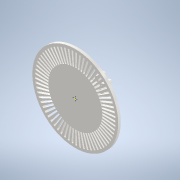
# Autodesk Inventor part: 正齿轮1
Saved by Autodesk Inventor 2020 (Build 240168000, 168)
## iProperties
CustomPartVersion: 1
Created: 2019-06-21
Part Number: 正齿轮1
Material: Steel
Document SubType Name: Modeling
Designer: User
Categories: <?xml version="1.0" encoding="UTF-16"?> <MemberInstance><Categories><FamilyTemplate><FamilyTemplateParameter ValueType="xs:double" Id="1" ObjectReferenceKey="da_z" ObjectType="kUserParameterObject"/><FamilyTemplateParameter ValueType="xs:double" Id="2" ObjectReferenceKey="da_b" ObjectType="kUserParameterObject"/><FamilyTemplateParameter ValueType="xs:double" Id="3" ObjectReferenceKey="da_beta" ObjectType="kUserParameterObject"/><FamilyTemplateParameter ValueType="xs:double" Id="4" ObjectReferenceKey="da_da" ObjectType="kUserParameterObject"/><FamilyTemplateParameter ValueType="xs:double" Id="5" ObjectReferenceKey="da_aw" ObjectType="kUserParameterObject"/><FamilyTemplateParameter ValueType="xs:string" Id="6" ObjectReferenceKey="EAIAABAAAACIAQAAAAAAAIAAAAAAAAAA" ObjectType="83910656" SubObjectId="SurfaceGeometry"/></FamilyTemplate><ParamToTemplateMap><ParamToTemplate CategoryParameter="//CategoryParameter[@InternalName='046C89C9-8512-4d59-83FE-43B91F4F132A']" TemplateParameter="1"/><ParamToTemplate CategoryParameter="//CategoryParameter[@InternalName='2552DF32-E462-4b46-AEBF-C6C7768E72AC']" TemplateParameter="2"/><ParamToTemplate CategoryParameter="//CategoryParameter[@InternalName='C9EE641D-15FC-4fae-A226-E94C4372FDD7']" TemplateParameter="3"/><ParamToTemplate><ParamToTemplate CategoryParameter="//CategoryParameter[@InternalName='00B6519A-459B-49c7-AD84-2E56D39A5744']" ConstantValue="0.104000"/></ParamToTemplate><ParamToTemplate><ParamToTemplate CategoryParameter="//CategoryParameter[@InternalName='04B31F0E-C7A6-4894-AA32-9629BEFACF47']" ConstantValue="1.000000"/></ParamToTemplate><ParamToTemplate><ParamToTemplate CategoryParameter="//CategoryParameter[@InternalName='43CBEC2E-7847-49e7-A936-2F7889FCB2D9']" ConstantValue="0.250000"/></ParamToTemplate><ParamToTemplate><ParamToTemplate CategoryParameter="//CategoryParameter[@InternalName='B1EFC894-105D-4ebd-86BF-FA20ED196853']" ConstantValue="0.333500"/></ParamToTemplate><ParamToTemplate><ParamToTemplate CategoryParameter="//CategoryParameter[@InternalName='51175063-3D10-4879-93E8-6246FE8B403D']" ConstantValue="2060000000.000000"/></ParamToTemplate><ParamToTemplate><ParamToTemplate CategoryParameter="//CategoryParameter[@InternalName='A3A52E27-4454-46a9-B0BD-C932399B70AF']" ConstantValue="0.300000"/></ParamToTemplate><ParamToTemplate><ParamToTemplate CategoryParameter="//CategoryParameter[@InternalName='91B76062-C214-41d9-B1B9-14D2AB99603D']" ConstantValue="0.080000"/></ParamToTemplate><ParamToTemplate><ParamToTemplate CategoryParameter="//CategoryParameter[@InternalName='374E806E-8B8A-4dda-A9AA-1039D6500AD2']" ConstantValue="12.500000"/></ParamToTemplate><ParamToTemplate><ParamToTemplate CategoryParameter="//CategoryParameter[@InternalName='2D373A89-B862-43d6-8D0B-0CBF12AB9F6C']" ConstantValue="0.349066"/></ParamToTemplate><ParamToTemplate CategoryParameter="//CategoryParameter[@InternalName='37777632-D6A2-4fac-9D53-DB8ACD95C989']" TemplateParameter="4"/><ParamToTemplate CategoryParameter="//CategoryParameter[@InternalName='FD1017F1-B727-4f7e-9707-0F86F1FF9423']" TemplateParameter="5"/><ParamToTemplate><ParamToTemplate CategoryParameter="//CategoryParameter[@InternalName='9E1B4470-B2D3-4ff1-B813-535BB4CDF51A']" ConstantValue="3520000.000000"/></ParamToTemplate><ParamToTemplate><ParamToTemplate CategoryParameter="//CategoryParameter[@InternalName='F8452263-BFF6-458c-9FB1-07C4B99E95CD']" ConstantValue="11400000.000000"/></ParamToTemplate><ParamToTemplate><ParamToTemplate CategoryParameter="//CategoryParameter[@InternalName='3E3BB259-FD49-497f-8171-6EBC954A3479']" ConstantValue="2.000000"/></ParamToTemplate><ParamToTemplate CategoryParameter="//CategoryParameter[@InternalName='27C3BAF2-7550-4e4b-AE2C-0DB134B7D9B7']" TemplateParameter="6"/></ParamToTemplateMap><Category DisplayName="Gear" InternalName="DC85795E-93AB-48d5-8EEE-5A27447B64BD" Mnemonic="Gear"><CategoryParameter DisplayName="z" InternalName="046C89C9-8512-4d59-83FE-43B91F4F132A" Mnemonic="z"/><CategoryParameter DisplayName="b" InternalName="2552DF32-E462-4b46-AEBF-C6C7768E72AC" Mnemonic="b"/><CategoryParameter DisplayName="||b|" InternalName="C9EE641D-15FC-4fae-A226-E94C4372FDD7" Mnemonic="beta"/><CategoryParameter DisplayName="x" InternalName="00B6519A-459B-49c7-AD84-2E56D39A5744" Mnemonic="x"/><CategoryParameter DisplayName="a*" InternalName="04B31F0E-C7A6-4894-AA32-9629BEFACF47" Mnemonic="a"/><CategoryParameter DisplayName="c*" InternalName="43CBEC2E-7847-49e7-A936-2F7889FCB2D9" Mnemonic="c"/><CategoryParameter DisplayName="r|.f|*" InternalName="B1EFC894-105D-4ebd-86BF-FA20ED196853" Mnemonic="rf"/><CategoryParameter DisplayName="E" InternalName="51175063-3D10-4879-93E8-6246FE8B403D" Mnemonic="E"/><CategoryParameter DisplayName="||m|" InternalName="A3A52E27-4454-46a9-B0BD-C932399B70AF" Mnemonic="mi"/><Category DisplayName="SpurGear" InternalName="26C5A22E-A91E-4dfd-A3B3-23CCAFAE1764" Mnemonic="SpurGear"><CategoryParameter DisplayName="m" InternalName="91B76062-C214-41d9-B1B9-14D2AB99603D" Mnemonic="m"/><CategoryParameter DisplayName="P" InternalName="374E806E-8B8A-4dda-A9AA-1039D6500AD2" Mnemonic="PP"/><CategoryParameter DisplayName="||a|" InternalName="2D373A89-B862-43d6-8D0B-0CBF12AB9F6C" Mnemonic="alpha"/><CategoryParameter DisplayName="d|.a|" InternalName="37777632-D6A2-4fac-9D53-DB8ACD95C989" Mnemonic="da"/><CategoryParameter DisplayName="a|.w|" InternalName="FD1017F1-B727-4f7e-9707-0F86F1FF9423" Mnemonic="aw"/><CategoryParameter DisplayName="||s||.Flim|" InternalName="9E1B4470-B2D3-4ff1-B813-535BB4CDF51A" Mnemonic="sFlim"/><CategoryParameter DisplayName="||s||.Hlim|" InternalName="F8452263-BFF6-458c-9FB1-07C4B99E95CD" Mnemonic="sHlim"/><CategoryParameter DisplayName="类型" InternalName="3E3BB259-FD49-497f-8171-6EBC954A3479" Mnemonic="type"/><CategoryParameter DisplayName="PitchDiameter" InternalName="27C3BAF2-7550-4e4b-AE2C-0DB134B7D9B7" Mnemonic="IDS_PITCHDIAM"/></Category></Category></Categories></MemberInstance>
Density: 1 g/cm^3
Appearance: Steel
Author: User
Autodesk Inventor part; units mm, degrees
sketch "Sketch1" plane through (0, 0, 0) normal (0, 0, 1) x (1, 0, 0)
  circle A0 centre (0, 0) radius 3.2554
  dimension "d0" = 6.5107
  constraints: 1 centre point
  measures "d0" diameter of A0
extrude "Extrusion1" add sketch "Sketch1" along normal blind 3
ref_plane "Work Plane2" through (0, 0, 1.5) normal (0, 0, 1) x (1, 0, 0)
sketch "Sketch2" plane through (0, 0, 0) normal (0, 0, -1) x (-1, 0, 0)
  circle A0 centre (0, 0) radius 3.2554 projected
  circle A1 centre (0, 0) radius 2.4643
  dimension "d3" = 4.9286
  constraints: 1 centre point, 1 coincident
  measures "d3" diameter of A1
surface extrude "中径" sketch "Sketch2" against normal through all shown no curves A1
ref_plane "Work Plane8" through (0, 0, 0) normal (0.8660254, 0.5, 0) x (0, 0, 1)
ref_plane "Work Plane9" through (0, 0, 0) normal (1, 0, 0) x (0, 1, 0)
spur gear teeth "正齿轮" teeth 6 pitch diameter 4.8 tip diameter 6.5107 root diameter 2.9664 face width 3 start plane through (0, 0, 0) normal (0, 0, -1) x (-1, 0, 0)
sketch "草图3" plane through (0, 0, 3) normal (0, 0, 1) x (1, 0, 0)
  circle A0 centre (0, 0) radius 1.5
  dimension "d49" = 3
  constraints: 1 centre point, 1 coincident
  measures "d49" diameter of A0
extrude "拉伸2" add sketch "草图3" along normal blind 7
sketch "草图4" plane through (0, 0, 10) normal (0, 0, 1) x (1, 0, 0)
  circle A0 centre (0, 0) radius 16
  line L0 (15, 0.3) -> (10, 0.3)
  line L1 (10, 0.3) -> (10, -0.3)
  line L2 (10, -0.3) -> (15, -0.3)
  line L3 (15, -0.3) -> (15, 0.3)
  line L4 (0, 0) -> (21.4745, 0)
  line L5 (14.901, 1.7463) -> (9.9244, 1.2637)
  line L6 (9.9823, 0.6665) -> (14.9589, 1.1491)
  line L7 (14.9589, 1.1491) -> (14.901, 1.7463)
  line L8 (9.9244, 1.2637) -> (9.9823, 0.6665)
  line L9 (14.6629, 3.1763) -> (9.7561, 2.2157)
  line L10 (9.8713, 1.6269) -> (14.7782, 2.5875)
  line L11 (14.7782, 2.5875) -> (14.6629, 3.1763)
  line L12 (9.7561, 2.2157) -> (9.8713, 1.6269)
  line L13 (14.2879, 4.5767) -> (9.4967, 3.1469)
  line L14 (9.6682, 2.572) -> (14.4595, 4.0017)
  line L15 (14.4595, 4.0017) -> (14.2879, 4.5767)
  line L16 (9.4967, 3.1469) -> (9.6682, 2.572)
  line L17 (13.7795, 5.9343) -> (9.1486, 4.0488)
  line L18 (9.3749, 3.4931) -> (14.0057, 5.3786)
  line L19 (14.0057, 5.3786) -> (13.7795, 5.9343)
  line L20 (9.1486, 4.0488) -> (9.3749, 3.4931)
  line L21 (13.1424, 7.2365) -> (8.7151, 4.9129)
  line L22 (8.994, 4.3816) -> (13.4213, 6.7052)
  line L23 (13.4213, 6.7052) -> (13.1424, 7.2365)
  line L24 (8.7151, 4.9129) -> (8.994, 4.3816)
  line L25 (12.3826, 8.4711) -> (8.2003, 5.7311)
  line L26 (8.5291, 5.2292) -> (12.7115, 7.9692)
  line L27 (12.7115, 7.9692) -> (12.3826, 8.4711)
  line L28 (8.2003, 5.7311) -> (8.5291, 5.2292)
  line L29 (11.5073, 9.6267) -> (7.6089, 6.4958)
  line L30 (7.9846, 6.0279) -> (11.883, 9.1589)
  line L31 (11.883, 9.1589) -> (11.5073, 9.6267)
  line L32 (7.6089, 6.4958) -> (7.9846, 6.0279)
  line L33 (10.5244, 10.6924) -> (6.9464, 7.1998)
  line L34 (7.3655, 6.7704) -> (10.9435, 10.263)
  line L35 (10.9435, 10.263) -> (10.5244, 10.6924)
  line L36 (6.9464, 7.1998) -> (7.3655, 6.7704)
  line L37 (9.4433, 11.6582) -> (6.2191, 7.8366)
  line L38 (6.6777, 7.4497) -> (9.9019, 11.2713)
  line L39 (9.9019, 11.2713) -> (9.4433, 11.6582)
  line L40 (6.2191, 7.8366) -> (6.6777, 7.4497)
  line L41 (8.2741, 12.5152) -> (5.4338, 8.4003)
  line L42 (5.9275, 8.0594) -> (8.7679, 12.1743)
  line L43 (8.7679, 12.1743) -> (8.2741, 12.5152)
  line L44 (5.4338, 8.4003) -> (5.9275, 8.0594)
  line L45 (7.0276, 13.2553) -> (4.5976, 8.8855)
  line L46 (5.122, 8.5939) -> (7.5519, 12.9637)
  line L47 (7.5519, 12.9637) -> (7.0276, 13.2553)
  line L48 (4.5976, 8.8855) -> (5.122, 8.5939)
  line L49 (5.7154, 13.8717) -> (3.7186, 9.2877)
  line L50 (4.2687, 9.0481) -> (6.2655, 13.6321)
  line L51 (6.2655, 13.6321) -> (5.7154, 13.8717)
  line L52 (3.7186, 9.2877) -> (4.2687, 9.0481)
  line L53 (4.3499, 14.3586) -> (2.8049, 9.6033)
  line L54 (3.3755, 9.4179) -> (4.9206, 14.1731)
  line L55 (4.9206, 14.1731) -> (4.3499, 14.3586)
  line L56 (2.8049, 9.6033) -> (3.3755, 9.4179)
  line L57 (2.9438, 14.7114) -> (1.8649, 9.8291)
  line L58 (2.4508, 9.6997) -> (3.5297, 14.5819)
  line L59 (3.5297, 14.5819) -> (2.9438, 14.7114)
  line L60 (1.8649, 9.8291) -> (2.4508, 9.6997)
  line L61 (1.5102, 14.9268) -> (0.9076, 9.9632)
  line L62 (1.5032, 9.8909) -> (2.1059, 14.8545)
  line L63 (2.1059, 14.8545) -> (1.5102, 14.9268)
  line L64 (0.9076, 9.9632) -> (1.5032, 9.8909)
  line L65 (0.0625, 15.0029) -> (-0.0583, 10.0043)
  line L66 (0.5415, 9.9898) -> (0.6624, 14.9884)
  line L67 (0.6624, 14.9884) -> (0.0625, 15.0029)
  line L68 (-0.0583, 10.0043) -> (0.5415, 9.9898)
  line L69 (-1.3857, 14.9389) -> (-1.0236, 9.952)
  line L70 (-0.4251, 9.9955) -> (-0.7873, 14.9823)
  line L71 (-0.7873, 14.9823) -> (-1.3857, 14.9389)
  line L72 (-1.0236, 9.952) -> (-0.4251, 9.9955)
  line L73 (-2.8211, 14.7354) -> (-1.9793, 9.8068)
  line L74 (-1.3879, 9.9078) -> (-2.2296, 14.8364)
  line L75 (-2.2296, 14.8364) -> (-2.8211, 14.7354)
  line L76 (-1.9793, 9.8068) -> (-1.3879, 9.9078)
  line L77 (-4.2301, 14.3943) -> (-2.9165, 9.5699)
  line L78 (-2.3376, 9.7276) -> (-3.6511, 14.5519)
  line L79 (-3.6511, 14.5519) -> (-4.2301, 14.3943)
  line L80 (-2.9165, 9.5699) -> (-2.3376, 9.7276)
  line L81 (-5.5996, 13.9189) -> (-3.8266, 9.2438)
  line L82 (-3.2655, 9.4565) -> (-5.0386, 14.1316)
  line L83 (-5.0386, 14.1316) -> (-5.5996, 13.9189)
  line L84 (-3.8266, 9.2438) -> (-3.2655, 9.4565)
  line L85 (-6.9168, 13.3134) -> (-4.7008, 8.8313)
  line L86 (-4.163, 9.0972) -> (-6.3789, 13.5794)
  line L87 (-6.3789, 13.5794) -> (-6.9168, 13.3134)
  line L88 (-4.7008, 8.8313) -> (-4.163, 9.0972)
  line L89 (-8.1694, 12.5837) -> (-5.5312, 8.3364)
  line L90 (-5.0216, 8.653) -> (-7.6598, 12.9003)
  line L91 (-7.6598, 12.9003) -> (-8.1694, 12.5837)
  line L92 (-5.5312, 8.3364) -> (-5.0216, 8.653)
  line L93 (-9.3458, 11.7365) -> (-6.31, 7.7636)
  line L94 (-5.8333, 8.1279) -> (-8.8691, 12.1008)
  line L95 (-8.8691, 12.1008) -> (-9.3458, 11.7365)
  line L96 (-6.31, 7.7636) -> (-5.8333, 8.1279)
  line L97 (-10.4349, 10.7797) -> (-7.0298, 7.1184)
  line L98 (-6.5905, 7.527) -> (-9.9956, 11.1883)
  line L99 (-9.9956, 11.1883) -> (-10.4349, 10.7797)
  line L100 (-7.0298, 7.1184) -> (-6.5905, 7.527)
  line L101 (-11.4266, 9.7223) -> (-7.684, 6.4067)
  line L102 (-7.2862, 6.8558) -> (-11.0287, 10.1714)
  line L103 (-11.0287, 10.1714) -> (-11.4266, 9.7223)
  line L104 (-7.684, 6.4067) -> (-7.2862, 6.8558)
  line L105 (-12.3116, 8.5741) -> (-8.2665, 5.6351)
  line L106 (-7.9138, 6.1206) -> (-11.9589, 9.0595)
  line L107 (-11.9589, 9.0595) -> (-12.3116, 8.5741)
  line L108 (-8.2665, 5.6351) -> (-7.9138, 6.1206)
  line L109 (-13.0816, 7.3458) -> (-8.7718, 4.811)
  line L110 (-8.4676, 5.3282) -> (-12.7775, 7.863)
  line L111 (-12.7775, 7.863) -> (-13.0816, 7.3458)
  line L112 (-8.7718, 4.811) -> (-8.4676, 5.3282)
  line L113 (-13.7295, 6.049) -> (-9.1952, 3.9419)
  line L114 (-8.9423, 4.4861) -> (-13.4767, 6.5931)
  line L115 (-13.4767, 6.5931) -> (-13.7295, 6.049)
  line L116 (-9.1952, 3.9419) -> (-8.9423, 4.4861)
  line L117 (-14.2492, 4.6956) -> (-9.5327, 3.0361)
  line L118 (-9.3335, 3.6021) -> (-14.0501, 5.2616)
  line L119 (-14.0501, 5.2616) -> (-14.2492, 4.6956)
  line L120 (-9.5327, 3.0361) -> (-9.3335, 3.6021)
  line L121 (-14.6359, 3.2985) -> (-9.7812, 2.1019)
  line L122 (-9.6376, 2.6844) -> (-14.4923, 3.881)
  line L123 (-14.4923, 3.881) -> (-14.6359, 3.2985)
  line L124 (-9.7812, 2.1019) -> (-9.6376, 2.6844)
  line L125 (-14.8859, 1.8705) -> (-9.9384, 1.148)
  line L126 (-9.8517, 1.7417) -> (-14.7992, 2.4642)
  line L127 (-14.7992, 2.4642) -> (-14.8859, 1.8705)
  line L128 (-9.9384, 1.148) -> (-9.8517, 1.7417)
  line L129 (-14.997, 0.4251) -> (-10.0028, 0.1835)
  line L130 (-9.9738, 0.7828) -> (-14.968, 1.0244)
  line L131 (-14.968, 1.0244) -> (-14.997, 0.4251)
  line L132 (-10.0028, 0.1835) -> (-9.9738, 0.7828)
  line L133 (-14.968, -1.0244) -> (-9.9738, -0.7828)
  line L134 (-10.0028, -0.1835) -> (-14.997, -0.4251)
  line L135 (-14.997, -0.4251) -> (-14.968, -1.0244)
  line L136 (-9.9738, -0.7828) -> (-10.0028, -0.1835)
  line L137 (-14.7992, -2.4642) -> (-9.8517, -1.7417)
  line L138 (-9.9384, -1.148) -> (-14.8859, -1.8705)
  line L139 (-14.8859, -1.8705) -> (-14.7992, -2.4642)
  line L140 (-9.8517, -1.7417) -> (-9.9384, -1.148)
  line L141 (-14.4923, -3.881) -> (-9.6376, -2.6844)
  line L142 (-9.7812, -2.1019) -> (-14.6359, -3.2985)
  line L143 (-14.6359, -3.2985) -> (-14.4923, -3.881)
  line L144 (-9.6376, -2.6844) -> (-9.7812, -2.1019)
  line L145 (-14.0501, -5.2616) -> (-9.3335, -3.6021)
  line L146 (-9.5327, -3.0361) -> (-14.2492, -4.6956)
  line L147 (-14.2492, -4.6956) -> (-14.0501, -5.2616)
  line L148 (-9.3335, -3.6021) -> (-9.5327, -3.0361)
  line L149 (-13.4767, -6.5931) -> (-8.9423, -4.4861)
  line L150 (-9.1952, -3.9419) -> (-13.7295, -6.049)
  line L151 (-13.7295, -6.049) -> (-13.4767, -6.5931)
  line L152 (-8.9423, -4.4861) -> (-9.1952, -3.9419)
  line L153 (-12.7775, -7.863) -> (-8.4676, -5.3282)
  line L154 (-8.7718, -4.811) -> (-13.0816, -7.3458)
  line L155 (-13.0816, -7.3458) -> (-12.7775, -7.863)
  line L156 (-8.4676, -5.3282) -> (-8.7718, -4.811)
  line L157 (-11.9589, -9.0595) -> (-7.9138, -6.1206)
  line L158 (-8.2665, -5.6351) -> (-12.3116, -8.5741)
  line L159 (-12.3116, -8.5741) -> (-11.9589, -9.0595)
  line L160 (-7.9138, -6.1206) -> (-8.2665, -5.6351)
  line L161 (-11.0287, -10.1714) -> (-7.2862, -6.8558)
  line L162 (-7.684, -6.4067) -> (-11.4266, -9.7223)
  line L163 (-11.4266, -9.7223) -> (-11.0287, -10.1714)
  line L164 (-7.2862, -6.8558) -> (-7.684, -6.4067)
  line L165 (-9.9956, -11.1883) -> (-6.5905, -7.527)
  line L166 (-7.0298, -7.1184) -> (-10.4349, -10.7797)
  line L167 (-10.4349, -10.7797) -> (-9.9956, -11.1883)
  line L168 (-6.5905, -7.527) -> (-7.0298, -7.1184)
  line L169 (-8.8691, -12.1008) -> (-5.8333, -8.1279)
  line L170 (-6.31, -7.7636) -> (-9.3458, -11.7365)
  line L171 (-9.3458, -11.7365) -> (-8.8691, -12.1008)
  line L172 (-5.8333, -8.1279) -> (-6.31, -7.7636)
  line L173 (-7.6598, -12.9003) -> (-5.0216, -8.653)
  line L174 (-5.5312, -8.3364) -> (-8.1694, -12.5837)
  line L175 (-8.1694, -12.5837) -> (-7.6598, -12.9003)
  line L176 (-5.0216, -8.653) -> (-5.5312, -8.3364)
  line L177 (-6.3789, -13.5794) -> (-4.163, -9.0972)
  line L178 (-4.7008, -8.8313) -> (-6.9168, -13.3134)
  line L179 (-6.9168, -13.3134) -> (-6.3789, -13.5794)
  line L180 (-4.163, -9.0972) -> (-4.7008, -8.8313)
  line L181 (-5.0386, -14.1316) -> (-3.2655, -9.4565)
  line L182 (-3.8266, -9.2438) -> (-5.5996, -13.9189)
  line L183 (-5.5996, -13.9189) -> (-5.0386, -14.1316)
  line L184 (-3.2655, -9.4565) -> (-3.8266, -9.2438)
  line L185 (-3.6511, -14.5519) -> (-2.3376, -9.7276)
  line L186 (-2.9165, -9.5699) -> (-4.2301, -14.3943)
  line L187 (-4.2301, -14.3943) -> (-3.6511, -14.5519)
  line L188 (-2.3376, -9.7276) -> (-2.9165, -9.5699)
  line L189 (-2.2296, -14.8364) -> (-1.3879, -9.9078)
  line L190 (-1.9793, -9.8068) -> (-2.8211, -14.7354)
  line L191 (-2.8211, -14.7354) -> (-2.2296, -14.8364)
  line L192 (-1.3879, -9.9078) -> (-1.9793, -9.8068)
  line L193 (-0.7873, -14.9823) -> (-0.4251, -9.9955)
  line L194 (-1.0236, -9.952) -> (-1.3857, -14.9389)
  line L195 (-1.3857, -14.9389) -> (-0.7873, -14.9823)
  line L196 (-0.4251, -9.9955) -> (-1.0236, -9.952)
  line L197 (0.6624, -14.9884) -> (0.5415, -9.9898)
  line L198 (-0.0583, -10.0043) -> (0.0625, -15.0029)
  line L199 (0.0625, -15.0029) -> (0.6624, -14.9884)
  line L200 (0.5415, -9.9898) -> (-0.0583, -10.0043)
  line L201 (2.1059, -14.8545) -> (1.5032, -9.8909)
  line L202 (0.9076, -9.9632) -> (1.5102, -14.9268)
  line L203 (1.5102, -14.9268) -> (2.1059, -14.8545)
  line L204 (1.5032, -9.8909) -> (0.9076, -9.9632)
  line L205 (3.5297, -14.5819) -> (2.4508, -9.6997)
  line L206 (1.8649, -9.8291) -> (2.9438, -14.7114)
  line L207 (2.9438, -14.7114) -> (3.5297, -14.5819)
  line L208 (2.4508, -9.6997) -> (1.8649, -9.8291)
  line L209 (4.9206, -14.1731) -> (3.3755, -9.4179)
  line L210 (2.8049, -9.6033) -> (4.3499, -14.3586)
  line L211 (4.3499, -14.3586) -> (4.9206, -14.1731)
  line L212 (3.3755, -9.4179) -> (2.8049, -9.6033)
  line L213 (6.2655, -13.6321) -> (4.2687, -9.0481)
  line L214 (3.7186, -9.2877) -> (5.7154, -13.8717)
  line L215 (5.7154, -13.8717) -> (6.2655, -13.6321)
  line L216 (4.2687, -9.0481) -> (3.7186, -9.2877)
  line L217 (7.5519, -12.9637) -> (5.122, -8.5939)
  line L218 (4.5976, -8.8855) -> (7.0276, -13.2553)
  line L219 (7.0276, -13.2553) -> (7.5519, -12.9637)
  line L220 (5.122, -8.5939) -> (4.5976, -8.8855)
  line L221 (8.7679, -12.1743) -> (5.9275, -8.0594)
  line L222 (5.4338, -8.4003) -> (8.2741, -12.5152)
  line L223 (8.2741, -12.5152) -> (8.7679, -12.1743)
  line L224 (5.9275, -8.0594) -> (5.4338, -8.4003)
  line L225 (9.9019, -11.2713) -> (6.6777, -7.4497)
  line L226 (6.2191, -7.8366) -> (9.4433, -11.6582)
  line L227 (9.4433, -11.6582) -> (9.9019, -11.2713)
  line L228 (6.6777, -7.4497) -> (6.2191, -7.8366)
  line L229 (10.9435, -10.263) -> (7.3655, -6.7704)
  line L230 (6.9464, -7.1998) -> (10.5244, -10.6924)
  line L231 (10.5244, -10.6924) -> (10.9435, -10.263)
  line L232 (7.3655, -6.7704) -> (6.9464, -7.1998)
  line L233 (11.883, -9.1589) -> (7.9846, -6.0279)
  line L234 (7.6089, -6.4958) -> (11.5073, -9.6267)
  line L235 (11.5073, -9.6267) -> (11.883, -9.1589)
  line L236 (7.9846, -6.0279) -> (7.6089, -6.4958)
  line L237 (12.7115, -7.9692) -> (8.5291, -5.2292)
  line L238 (8.2003, -5.7311) -> (12.3826, -8.4711)
  line L239 (12.3826, -8.4711) -> (12.7115, -7.9692)
  line L240 (8.5291, -5.2292) -> (8.2003, -5.7311)
  line L241 (13.4213, -6.7052) -> (8.994, -4.3816)
  line L242 (8.7151, -4.9129) -> (13.1424, -7.2365)
  line L243 (13.1424, -7.2365) -> (13.4213, -6.7052)
  line L244 (8.994, -4.3816) -> (8.7151, -4.9129)
  line L245 (14.0057, -5.3786) -> (9.3749, -3.4931)
  line L246 (9.1486, -4.0488) -> (13.7795, -5.9343)
  line L247 (13.7795, -5.9343) -> (14.0057, -5.3786)
  line L248 (9.3749, -3.4931) -> (9.1486, -4.0488)
  line L249 (14.4595, -4.0017) -> (9.6682, -2.572)
  line L250 (9.4967, -3.1469) -> (14.2879, -4.5767)
  line L251 (14.2879, -4.5767) -> (14.4595, -4.0017)
  line L252 (9.6682, -2.572) -> (9.4967, -3.1469)
  line L253 (14.7782, -2.5875) -> (9.8713, -1.6269)
  line L254 (9.7561, -2.2157) -> (14.6629, -3.1763)
  line L255 (14.6629, -3.1763) -> (14.7782, -2.5875)
  line L256 (9.8713, -1.6269) -> (9.7561, -2.2157)
  line L257 (14.9589, -1.1491) -> (9.9823, -0.6665)
  line L258 (9.9244, -1.2637) -> (14.901, -1.7463)
  line L259 (14.901, -1.7463) -> (14.9589, -1.1491)
  line L260 (9.9823, -0.6665) -> (9.9244, -1.2637)
  dimension "d52" = 32
  dimension "d53" = 0.6
  dimension "d54" = 15
  dimension "d55" = 5
  dimension "d58" = 360
  constraints: 522 end point, 3 horizontal, 2 parallel, 1 centre point, 1 coincident, 1 perpendicular, 1 symmetric about line, 521 other
  measures "d52" diameter of A0
  measures "d53" distance of L0.end L1.end
  measures "d54" distance from line of L3 L4.start
  measures "d55" distance of L1.end L2.end
extrude "拉伸3" add sketch "草图4" along normal blind 1
sketch "草图5" plane through (0, 0, 11) normal (0, 0, 1) x (1, 0, 0)
  point P0 (0, 0)
  point P1 (0, 0)
  constraints: 1 coincident
equation "\"d0\" = da_da"
equation "\"d1\" = da_b"
equation "\"d3\" = da_dw"
equation "\"d16\" = da_aw"
equation "\"d43\" = da_aw"
equation "\"d46\" = da_aw"
equation "\"da_da\" = 6.510702"
equation "\"da_b\" = 3"
equation "\"da_dw\" = 4.928571"
equation "\"da_aw\" = 11.5"
body "Solid1"
body "Srf1"
